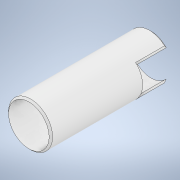
# Autodesk Inventor part: hull_mid
Saved by Autodesk Inventor 2020.1 (Build 241239000, 239)
## iProperties
Created: 2019-11-08
Part Number: hull_mid
Material: PVC-Piping
Document SubType Name: Modeling
Designer: agmle
Mass: 4589.86 g
Surface Area: 7708.26 cm^2
Volume: 3278.47 cm^3
Density: 1.4 g/cm^3
Appearance: Smooth - White
Author: agmle
Autodesk Inventor part; units mm, degrees
ref_plane "YZ Plane" through (0, 0, 0) normal (1, 0, 0) x (0, 1, 0)
ref_plane "XZ Plane" through (0, 0, 0) normal (0, 1, 0) x (-1, 0, 0)
ref_plane "XY Plane" through (0, 0, 0) normal (0, 0, 1) x (1, 0, 0)
sketch "Sketch1" plane through (0, 0, 0) normal (0, 0, 1) x (1, 0, 0)
  circle A0 centre (0, 0) radius 109.5375
  circle A1 centre (0, 0) radius 100.8634
  dimension "d0" = 219.075
  dimension "d1" = 8.6741
  constraints: 2 centre point, 2 coincident
  measures "d0" diameter of A0
  measures "d1" radial gap between concentric circles of A0 A1
extrude "Extrusion1" add sketch "Sketch1" along normal blind 609.6
sketch "Sketch2" plane through (0, 0, 0) normal (0, 0, -1) x (-1, 0, 0)
  line L0 (-74.8778, 79.9486) -> (-109.5375, 79.9486)
  line L1 (-109.5375, 79.9486) -> (-109.5375, -79.9486)
  line L2 (-109.5375, -79.9486) -> (-74.8778, -79.9486)
  line L3 (-74.8778, -79.9486) -> (-74.8778, 79.9486)
  circle A0 centre (0, 0) radius 109.5375 construction
  dimension "d4" = 34.6597
  constraints: 8 end point, 2 parallel, 2 point on circle, 1 horizontal, 1 perpendicular, 1 tangent
  measures "d4" distance of L0.start L0.end
extrude "Extrusion2" cut sketch "Sketch2" against normal blind 152.4
chamfer "Chamfer1" distance 8.6741 angle 45 2 edges at (-109.5375, 0, 609.6) (-109.5375, 0, 0)
equation "\"d0\" = hull_od"
equation "\"d1\" = hull_wall"
equation "\"d2\" = hull_length"
equation "\"d4\" = slab_thick"
equation "\"d5\" = 2 * impeller_od"
equation "\"d8\" = hull_wall"
equation "\"hull_od\" = 219.075"
equation "\"hull_id\" = 201.7268"
equation "\"hull_wall\" = 8.6741"
equation "\"hull_length\" = 609.6"
equation "\"hull_spacing\" = 390.525"
equation "\"impeller_od\" = 76.2"
equation "\"impeller_clearance\" = 0.5"
equation "\"impeller_shaft_id\" = 3.175"
equation "\"impeller_shaft_od\" = 5.715"
equation "\"impeller_shaft_support\" = 3.175"
equation "\"impeller_intake_od\" = 19.05"
equation "\"impeller_vane_thick\" = 2"
equation "\"impeller_vane_inner_rad\" = 3.175"
equation "\"impeller_vane_outer_rad\" = 0.37206"
equation "\"magnet_od\" = 5.95"
equation "\"magnet_clearance\" = 0.25"
equation "\"magnet_rad\" = 0.25"
equation "\"magnet_circle_offset\" = 3.175"
equation "\"motor_shaft_od\" = 12.7"
equation "\"motor_shaft_length\" = 31.75"
equation "\"motor_shaft_key\" = 3.048"
equation "\"slab_thick\" = 34.659725"
body "Solid1"
